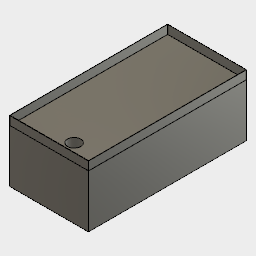
Ladefläche (Autodesk Fusion 360 design; units mm, degrees)
Autodesk Fusion 360 part; units mm, degrees
box "Grundkörper Quader1" add length 180 width 90 height 70 placed x (0, 0, -1) y (-1, 0, 0) z (0, 1, 0) at (19.6846, 0, 34.8152)
box "Grundkörper Quader2" cut length 179.5 width 89.5 height -10 placed x (0, 0, -1) y (-1, 0, 0) z (0, 1, 0) at (19.5, 70, 34.5)
box "Grundkörper Quader3" cut length 170 width 80 height -40 placed x (0, 0, 1) y (-1, 0, 0) z (0, -1, 0) at (15, 0, -140)
hole "Bohrung1" at (-16.4163, 60, 15.0098) direction (0, -1, 0) diameter 15 depth 40 tip angle 180
